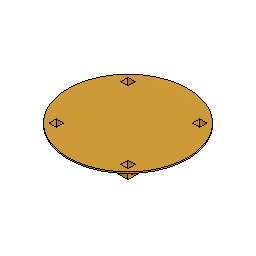
Plateau_1 (Autodesk Fusion 360 design; units mm, degrees)
Autodesk Fusion 360 part; units mm, degrees
sketch "Sketch1" plane through (0, 0, 0) normal (0, 0, 1) x (1, 0, 0)
  line L0 (82.6, -82.6) -> (67.4, -82.6)
  line L1 (-67.4, 67.4) -> (-82.6, 82.6) construction
  line L2 (82.6, 82.6) -> (82.6, 67.4)
  line L3 (67.4, -67.4) -> (82.6, -67.4)
  line L4 (82.6, 67.4) -> (67.4, 67.4)
  circle A0 centre (75, -75) radius 2.1
  line L5 (-67.4, -82.6) -> (-82.6, -82.6)
  circle A1 centre (0, 0) radius 125
  line L6 (67.4, 82.6) -> (82.6, 82.6)
  line L7 (-67.4, -67.4) -> (-67.4, -82.6)
  line L8 (-67.4, 82.6) -> (-67.4, 67.4)
  line L9 (82.6, -67.4) -> (82.6, -82.6)
  circle A2 centre (-75, 75) radius 2.1
  line L10 (-82.6, -82.6) -> (-82.6, -67.4)
  line L11 (-82.6, 67.4) -> (-82.6, 82.6)
  line L12 (-82.6, -67.4) -> (-67.4, -67.4)
  circle A3 centre (-75, -75) radius 2.1
  line L13 (-82.6, 82.6) -> (-67.4, 82.6)
  line L14 (-67.4, 67.4) -> (-82.6, 67.4)
  circle A4 centre (75, 75) radius 2.1
  line L15 (-82.6, 67.4) -> (-67.4, 82.6) construction
  line L16 (0, 0) -> (0, 43.6885) construction
  line L17 (67.4, 67.4) -> (67.4, 82.6)
  line L18 (0, 0) -> (-31.7204, 0) construction
  line L19 (67.4, -82.6) -> (67.4, -67.4)
  line L20 (-65.4, 84.6) -> (-65.4, 65.4)
  line L21 (-65.4, 65.4) -> (-84.6, 65.4)
  line L22 (-84.6, 65.4) -> (-84.6, 84.6)
  line L23 (-84.6, 84.6) -> (-65.4, 84.6)
  line L24 (84.6, 84.6) -> (84.6, 65.4)
  line L25 (65.4, 84.6) -> (84.6, 84.6)
  line L26 (84.6, 65.4) -> (65.4, 65.4)
  line L27 (65.4, 65.4) -> (65.4, 84.6)
  line L28 (-65.4, -65.4) -> (-65.4, -84.6)
  line L29 (-84.6, -65.4) -> (-65.4, -65.4)
  line L30 (-65.4, -84.6) -> (-84.6, -84.6)
  line L31 (-84.6, -84.6) -> (-84.6, -65.4)
  line L32 (84.6, -65.4) -> (84.6, -84.6)
  line L33 (65.4, -65.4) -> (84.6, -65.4)
  line L34 (84.6, -84.6) -> (65.4, -84.6)
  line L35 (65.4, -84.6) -> (65.4, -65.4)
  point P0 (-75, 75)
  dimension "d3" = 150
  dimension "d4" = -150
  dimension "d7" = 150
  dimension "d8" = -150
  dimension "d9" = 15.2
  dimension "d10" = 15.2
  dimension "d11" = 75
  dimension "d12" = 75
  dimension "d13" = 250
  dimension "d16" = 4.2
  dimension "d15" = -2
  constraint horizontal L14
  constraint perpendicular L11 L14
  constraint parallel L13 L14
  constraint parallel L8 L11
  constraint coincident P0 L1
  constraint coincident P0 L15
  constraint coincident A1.centre L16.start
  constraint perpendicular L13 L16
  constraint perpendicular L16 L18
  constraint coincident P0 A2.centre
  measures "d9" distance of L1.end L8.start
  measures "d10" distance of L11.start L1.end
  measures "d11" vertical distance of A1.centre P0
  measures "d12" horizontal distance of A1.centre P0
  measures "d13" diameter of A1
  measures "d16" diameter of A2
extrude "Extrude1" add sketch "Sketch1" along normal blind 3 contours A1 | L20 L21 L22 L23 | L24 L25 L26 L27 | L28 L29 L30 L31 | L32 L33 L34 L35
extrude "Extrude2" add sketch "Sketch1" against normal blind 15 contours L20 L21 L22 L23 | L24 L25 L26 L27 | L28 L29 L30 L31 | L32 L33 L34 L35
fillet "Fillet2" radius 4 16 edges at (-75, -84.6, 0) (-65.4, -75, 0) (75, -84.6, 0) (84.6, -75, 0) (-75, 65.4, 0) (-65.4, 75, 0) (75, 65.4, 0) (84.6, 75, 0) (-84.6, -75, 0) (-75, -65.4, 0) (65.4, -75, 0) (75, -65.4, 0) (-84.6, 75, 0) (-75, 84.6, 0) (65.4, 75, 0) (75, 84.6, 0)
sketch "Sketch2" plane through (84.6, 0, 0) normal (1, 0, 0) x (0, 1, 0)
  line L0 (-65.4, -15) -> (-65.4, -4)
  line L1 (-84.6, -15) -> (-65.4, -15)
  line L2 (-84.6, -4) -> (-84.6, -15)
  line L3 (-84.6, -4) -> (-65.4, -15) construction
  line L4 (84.6, -15) -> (84.6, -4)
  line L5 (65.4, -15) -> (84.6, -15)
  line L6 (65.4, -4) -> (65.4, -15)
  line L7 (65.4, -4) -> (84.6, -15) construction
  circle A0 centre (-75, -9.5) radius 1.6
  circle A1 centre (75, -9.5) radius 1.6
  line L8 (-65.4, -4) -> (-84.6, -4)
  line L9 (84.6, -4) -> (65.4, -4)
  dimension "d24" = 3.2
  dimension "d25" = 3.2
  constraint coincident L2.start L3.start
  constraint coincident L0.start L1.end
  constraint coincident L6.start L7.start
  constraint coincident L4.start L5.end
  constraint midpoint L3 A0.centre
  constraint midpoint L7 A1.centre
  measures "d24" diameter of A0
  measures "d25" diameter of A1
extrude "Extrude3" cut sketch "Sketch2" against normal through all contours A0 | A1
ref_plane "WorkPlane1" through (55, 0, 0) normal (1, 0, 0) x (0, 1, 0)
split "Split1" [suppressed]
ref_plane "WorkPlane2" through (0, -55, 0) normal (0, 1, 0) x (0, 0, 1)
split "Split2" [suppressed]
named bodies: "Plateau_1"
